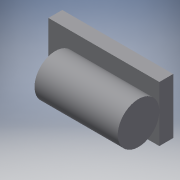
# Autodesk Inventor part: Part41
Saved by Autodesk Inventor 2016 (Build 200138000, 138)
## iProperties
Created: 2016-01-27
Part Number: Part41
Material: Generic
Document SubType Name: Modeling
Designer: seve
Density: 1 g/cm^3
Appearance: Default
Author: seve
Autodesk Inventor part; units mm, degrees
ref_plane "YZ Plane" through (0, 0, 0) normal (1, 0, 0) x (0, 1, 0)
ref_plane "XZ Plane" through (0, 0, 0) normal (0, 1, 0) x (-1, 0, 0)
ref_plane "XY Plane" through (0, 0, 0) normal (0, 0, 1) x (1, 0, 0)
sketch "Sketch1" plane through (0, 0, 0) normal (0, 0, 1) x (1, 0, 0)
  circle A0 centre (0.0041, -0.0026) radius 0.7938 projected
  line L0 (-3.1151, -1.4952) -> (3.2349, -1.4952)
  line L1 (3.2349, -1.4952) -> (3.2349, 1.6798)
  line L2 (3.2349, 1.6798) -> (-3.1151, 1.6798)
  line L3 (-3.1151, 1.6798) -> (-3.1151, -1.4952)
  point P0 (0, 0)
  dimension "d0" = 6.35
  dimension "d1" = 3.175
  constraints: 8 end point, 2 parallel, 1 horizontal, 1 perpendicular
  measures "d0" distance of L1.end L2.end
  measures "d1" distance of L0.end L1.end
extrude "Extrusion1" add sketch "Sketch1" along normal blind 0.7937 contours A0 | L3 L2 L1 L0
sketch "Sketch2" plane through (3.2349, -1.4952, 0) normal (1, 0, 0) x (0, 0, -1)
  circle A0 centre (-1.9844, 1.7393) radius 1.1906
  line L0 (-0.7937, 0) -> (-0.7937, 3.175) projected
  point P0 (0, 1.4952)
  dimension "d4" = 2.3813
  constraints: 1 centre point, 1 tangent
  measures "d4" diameter of A0
extrude "Extrusion2" add sketch "Sketch2" against normal blind 4.7625
sketch "Sketch3" plane through (0, 0, 0.7937) normal (0, 0, 1) x (1, 0, 0)
  point P0 (0, 0)
body "Solid1"
